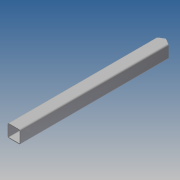
# Autodesk Inventor part: 2f2ax2
Saved by Autodesk Inventor 2014 SP1 (Build 180222100, 222)
## iProperties
Company: HERA Project
Created: 2013-06-27
Part Number: 2f2ax2
Material: Steel
Description: Feed backplane support interior piece 2
Document SubType Name: Modeling
Designer: David DeBoer
Mass: 176.671 g
Surface Area: 275.636 cm^2
Volume: 22.5058 cm^3
Density: 7.85 g/cm^3
Appearance: Steel
Title: Feed backplane support interior piece 2
Author: David DeBoer
Autodesk Inventor part; units mm, degrees
ref_plane "YZ Plane" through (0, 0, 0) normal (1, 0, 0) x (0, 1, 0)
ref_plane "XZ Plane" through (0, 0, 0) normal (0, 1, 0) x (-1, 0, 0)
ref_plane "XY Plane" through (0, 0, 0) normal (0, 0, 1) x (1, 0, 0)
sketch "Sketch1" plane through (0, 0, 0) normal (0, 0, 1) x (1, 0, 0)
  line L0 (3.7363, 0) -> (22.7863, 0)
  line L1 (25.9613, 3.175) -> (25.9613, 22.225)
  line L2 (22.7863, 25.4) -> (3.7363, 25.4)
  line L3 (0.5613, 22.225) -> (0.5613, 3.175)
  arc A0 (3.7363, 25.4) -> (0.5613, 22.225) centre (3.7363, 22.225) ccw
  arc A1 (0.5613, 3.175) -> (3.7363, 0) centre (3.7363, 3.175) ccw
  arc A2 (22.7863, 0) -> (25.9613, 3.175) centre (22.7863, 3.175) ccw
  arc A3 (25.9613, 22.225) -> (22.7863, 25.4) centre (22.7863, 22.225) ccw
  line L4 (3.7363, 23.749) -> (22.7863, 23.749)
  arc A4 (24.3103, 22.225) -> (22.7863, 23.749) centre (22.7863, 22.225) ccw
  line L5 (24.3103, 22.225) -> (24.3103, 3.175)
  arc A5 (22.7863, 1.651) -> (24.3103, 3.175) centre (22.7863, 3.175) ccw
  line L6 (22.7863, 1.651) -> (3.7363, 1.651)
  arc A6 (2.2123, 3.175) -> (3.7363, 1.651) centre (3.7363, 3.175) ccw
  line L7 (2.2123, 3.175) -> (2.2123, 22.225)
  arc A7 (3.7363, 23.749) -> (2.2123, 22.225) centre (3.7363, 22.225) ccw
  point P0 (0, 0)
  point P1 (0.5613, 0)
  point P2 (25.9613, 0)
  point P3 (0.5613, 25.4)
  dimension "d0" = 25.4
  dimension "d2" = 25.4
  dimension "d3" = 3.175
  dimension "d4" = 1.651
  constraints: 16 end point, 16 point on circle, 8 centre point, 8 tangent, 6 point on line, 4 parallel, 3 equal radius, 2 perpendicular, 1 horizontal, 7 other
  measures "d0" distance of point (0.561, 0) point (25.961, 0)
  measures "d2" distance of point (0.561, 25.4) point (0.561, 0)
  measures "d3" radius of A0
  measures "d4" distance between parallel lines of L4 L2
extrude "Extrusion1" add sketch "Sketch1" along normal blind 304.8
sketch "Sketch2" plane through (3.7363, 25.4, 0) normal (0, 1, 0) x (1, 0, 0)
  line L0 (22.2338, 0) -> (22.2338, -14.667)
  line L1 (19.05, -304.8) -> (0, -304.8) projected
  line L2 (9.525, -162.56) -> (9.525, -304.8) construction
  line L3 (-3.1838, 0) -> (-3.1838, -14.667)
  line L4 (9.525, -7.33) -> (22.2338, -14.667)
  line L5 (9.525, -7.33) -> (-3.1838, -14.667)
  line L6 (-3.1838, 0) -> (22.2338, 0)
  point P0 (-3.7363, 0)
  constraints: 12 end point, 2 symmetric about line, 1 midpoint, 1 perpendicular
extrude "Extrusion3" cut sketch "Sketch2" against normal blind 25.4
body "Solid1"
